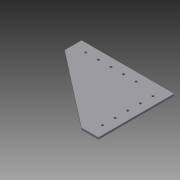
# Autodesk Inventor part: no_cutout_bracket_top(ncbt)
Saved by Autodesk Inventor 2015 SP1 (Build 190203100, 203)
## iProperties
Created: 2015-10-09
Part Number: no_cutout_bracket_top(ncbt)
Material: Generic
Document SubType Name: Sheet Metal
Designer: elilitwack
Density: 1 g/cm^3
Sheet Metal Rule: Default
Appearance: Default
Author: elilitwack
Autodesk Inventor part; units mm, degrees
ref_plane "YZ Plane" through (0, 0, 0) normal (1, 0, 0) x (0, 1, 0)
ref_plane "XZ Plane" through (0, 0, 0) normal (0, 1, 0) x (-1, 0, 0)
ref_plane "XY Plane" through (0, 0, 0) normal (0, 0, 1) x (1, 0, 0)
sketch "face_sketch" plane through (0, 0, 0) normal (0, 1, 0) x (-1, 0, 0)
  line L0 (0, 0) -> (0, -114.3)
  line L1 (139.7, -114.3) -> (139.7, -88.9)
  line L2 (139.7, -88.9) -> (25.4, 0)
  line L3 (25.4, 0) -> (0, 0)
  line L4 (25.4, 0) -> (25.4, -114.3) construction
  line L5 (0, -114.3) -> (25.4, -114.3)
  line L6 (25.4, -114.3) -> (139.7, -114.3)
  dimension "d0" = 114.3
  dimension "d2" = 25.4
  dimension "d3" = 25.4
  dimension "d5" = 114.3
  constraints: 14 end point, 2 horizontal, 2 vertical, 1 parallel, 1 perpendicular
  measures "d0" distance of L0.start L0.end
  measures "d2" distance of L2.end L0.start
  measures "d3" distance of L1.start L1.end
  measures "d5" distance of L4.end L1.start
extrude "Plate1" add sketch "face_sketch" along normal blind 3.048
sketch "Sketch4" plane through (0, 3.048, 0) normal (0, 1, 0) x (1, 0, 0)
  line L0 (-25.4, 0) -> (0, 0) construction
  line L1 (-12.7, 0) -> (-12.7, 19.05) construction
  line L2 (-12.7, 19.05) -> (-12.7, 38.1) construction
  line L3 (-12.7, 38.1) -> (-12.7, 57.15) construction
  line L4 (-12.7, 57.15) -> (-12.7, 76.2) construction
  line L5 (-12.7, 76.2) -> (-12.7, 95.25) construction
  line L6 (-12.7, 95.25) -> (-12.7, 114.3) construction
  line L7 (0, 114.3) -> (-139.7, 114.3) construction
  line L8 (-139.7, 114.3) -> (-139.7, 88.9) construction
  line L9 (-139.7, 101.6) -> (-120.65, 101.6) construction
  line L10 (-120.65, 101.6) -> (-101.6, 101.6) construction
  line L11 (-101.6, 101.6) -> (-82.55, 101.6) construction
  line L12 (-82.55, 101.6) -> (-63.5, 101.6) construction
  line L13 (-63.5, 101.6) -> (-44.45, 101.6) construction
  line L14 (-44.45, 101.6) -> (-25.4, 101.6) construction
  line L15 (-25.4, 0) -> (-25.4, 101.6) construction
  constraints: 26 end point, 11 point on line, 10 coincident, 10 collinear, 2 midpoint, 2 vertical, 1 horizontal
hole "Hole1" at (-12.7, 3.048, -19.05) at (-12.7, 3.048, -38.1) at (-12.7, 3.048, -57.15) at (-12.7, 3.048, -76.2) at (-12.7, 3.048, -95.25) at (-120.65, 3.048, -101.6) at (-101.6, 3.048, -101.6) at (-82.55, 3.048, -101.6) at (-63.5, 3.048, -101.6) at (-44.45, 3.048, -101.6) direction (0, -1, 0) diameter 3.5719 depth 3.048 tip angle 118
equation "\"d6\" = rv_hole_diameter"
equation "\"d11\" = Thickness"
equation "\"d0\" = ncbt_rivet_row_length"
equation "\"d2\" = st_outer_diameter"
equation "\"d3\" = st_outer_diameter"
equation "\"d5\" = ncbt_rivet_row_length"
equation "\"BendRadius\" = Thickness"
equation "\"BendReliefWidth\" = Thickness"
equation "\"BendReliefDepth\" = 0.5 * Thickness"
equation "\"CornerReliefSize\" = 4 * Thickness"
equation "\"MinimumRemnant\" = 2 * Thickness"
equation "\"TransitionRadius\" = BendRadius"
equation "\"JacobiRadiusSize\" = BendRadius"
equation "\"GapSize\" = Thickness"
equation "\"bp_thickness\" = 3.048"
equation "\"bp_height\" = 25.4"
equation "\"bp_width\" = 25.4"
equation "\"bp_axle_height\" = 25.4"
equation "\"magic_axle_offset\" = 3.175"
equation "\"bp_tensioner_width\" = 6.35"
equation "\"bp_tensioner_height\" = 19.05"
equation "\"bp_tensioner_from_bottom\" = 50.8"
equation "\"bp_tensioner_from_side\" = 25.4"
equation "\"bp_tensioner_wood_mount_from_tensioner_top\" = 12.7"
equation "\"bp_tensioner_wood_mount_diameter\" = 6.35"
equation "\"gb_mh_seperation\" = 111.1504"
equation "\"gb_mh_diameter\" = 6.35"
equation "\"gb_axle_from_edge\" = 38.1"
equation "\"gb_width\" = 127"
equation "\"gb_bearing_diameter\" = 28.575"
equation "\"gb_to_bottom_of_side_assembly\" = 4.7752"
equation "\"rivet_row_length\" = 114.3"
equation "\"rv_hole_diameter\" = 3.57187"
equation "\"st_outer_diameter\" = 25.4"
equation "\"st_wall_thickness\" = 6.35"
equation "\"st_length\" = 939.8"
equation "\"st_gbmh_from_center\" = 0.5 * gb_mh_seperation"
equation "\"st_cutout_depth_right\" = 254"
equation "\"st_cutout_depth_left\" = 254"
equation "\"st_rivet_distance\" = 19.05"
equation "\"so_inner_diameter\" = 6.35"
equation "\"so_wall_thickness\" = 3.048"
equation "\"so_length\" = 25.4"
equation "\"twb_width\" = st_outer_diameter"
equation "\"twb_length\" = bp_tensioner_width + 2 * twb_margin_on_each_side"
equation "\"twb_height\" = 2 * bp_tensioner_wood_mount_diameter + bp_tensioner_height + 2 * bp_tensioner_wood_mount_from_tensioner_top + twb_margin_on_each_side"
equation "\"twb_margin_on_each_side\" = 6.35"
equation "\"twb_tensioner_from_edge\" = -0.5 * bp_tensioner_height + 0.5 * twb_height"
equation "\"tb_rivet_row_length\" = 127"
equation "\"ncbt_rivet_row_length\" = 114.3"
equation "\"d4\" = BendRadius"
equation "\"Thickness\" = 3.048"
body "Solid1"
